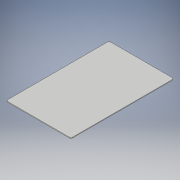
# Autodesk Inventor part: std credit card
Saved by Autodesk Inventor 2019.4 (Build 234330000, 330)
## iProperties
Created: 2020-11-10
Part Number: std credit card
Material: Generic
Document SubType Name: Modeling
Designer: caleb
Density: 1 g/cm^3
Appearance: Default
Author: caleb
Autodesk Inventor part; units mm, degrees
ref_plane "YZ Plane" through (0, 0, 0) normal (1, 0, 0) x (0, 1, 0)
ref_plane "XZ Plane" through (0, 0, 0) normal (0, 1, 0) x (-1, 0, 0)
ref_plane "XY Plane" through (0, 0, 0) normal (0, 0, 1) x (1, 0, 0)
sketch "Sketch1" plane through (0, 0, 0) normal (0, 1, 0) x (-1, 0, 0)
  line L0 (26.9875, 42.799) -> (-26.9875, 42.799)
  line L1 (-26.9875, 42.799) -> (-26.9875, -42.799)
  line L2 (-26.9875, -42.799) -> (26.9875, -42.799)
  line L3 (26.9875, -42.799) -> (26.9875, 42.799)
  point P0 (0, 0)
  dimension "d0" = 85.598
  dimension "d1" = 53.975
  dimension "d2" = 42.799
  dimension "d3" = 26.9875
  constraints: 8 end point, 2 parallel, 1 horizontal, 1 perpendicular
  measures "d0" distance of L2.end L0.start
  measures "d1" distance of L1.end L2.end
  measures "d2" distance from line of L0 point (0, 0)
  measures "d3" distance from line of L3 point (0, 0)
extrude "Extrusion1" add sketch "Sketch1" along normal blind 0.6096
fillet "Fillet1" radius 1.27 1 edges at (26.9875, 0.3048, 42.799)
fillet "Fillet2" radius 1.27 1 edges at (-26.9875, 0.3048, 42.799)
fillet "Fillet3" radius 1.27 2 edges at (-26.9875, 0.3048, -42.799) (26.9875, 0.3048, -42.799)
body "Solid1"
